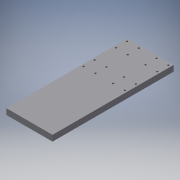
# Autodesk Inventor part: BLOCO_SUPORTE_EIXO_Z
Saved by Autodesk Inventor 2018 (Build 220112000, 112)
## iProperties
Created: 2018-10-10
Part Number: BLOCO_SUPORTE_EIXO_Z
Material: Genérico
Document SubType Name: Modeling
Designer: Georgines
Density: 1 g/cm^3
Appearance: Padrão
Author: Georgines
Autodesk Inventor part; units mm, degrees
ref_plane "YZ Plane" through (0, 0, 0) normal (1, 0, 0) x (0, 1, 0)
ref_plane "XZ Plane" through (0, 0, 0) normal (0, 1, 0) x (-1, 0, 0)
ref_plane "XY Plane" through (0, 0, 0) normal (0, 0, 1) x (1, 0, 0)
sketch "Esboço1" plane through (0, 0, 0) normal (0, 0, 1) x (1, 0, 0)
  line L0 (-20, 180.23) -> (105, 180.23)
  line L1 (105, 180.23) -> (105, -148.24)
  line L2 (105, -148.24) -> (-20, -148.24)
  line L3 (-20, -148.24) -> (-20, 180.23)
  dimension "d0" = 125
  dimension "d1" = 328.47
  constraints: 8 end point, 2 parallel, 1 horizontal, 1 perpendicular
  measures "d0" distance of L1.end L2.end
  measures "d1" distance of L0.end L1.end
extrude "Extrusão1" add sketch "Esboço1" along normal blind 15.88
sketch "Esboço3" plane through (0, 0, 0) normal (0, 0, -1) x (-1, 0, 0)
  circle A0 centre (-18.5, 54.73) radius 2.9 construction
  circle A1 centre (13.5, 54.73) radius 2.9 construction
  circle A2 centre (-66.5, 54.73) radius 2.9 construction
  circle A3 centre (-98.5, 54.73) radius 2.9 construction
  circle A4 centre (-98.5, 84.73) radius 2.9 construction
  circle A5 centre (-66.5, 84.73) radius 2.9 construction
  circle A6 centre (-18.5, 84.73) radius 2.9 construction
  circle A7 centre (13.5, 84.73) radius 2.9 construction
  circle A8 centre (-18.5, 172.73) radius 2.9 construction
  circle A9 centre (13.5, 172.73) radius 2.9 construction
  circle A10 centre (13.5, 142.73) radius 2.9 construction
  circle A11 centre (-18.5, 142.73) radius 2.9 construction
  circle A12 centre (-66.5, 172.73) radius 2.9 construction
  circle A13 centre (-98.5, 172.73) radius 2.9 construction
  circle A14 centre (-98.5, 142.73) radius 2.9 construction
  circle A15 centre (-66.5, 142.73) radius 2.9 construction
  point P0 (0, 0)
  constraints: 16 centre point
hole "Furo1" at (66.5, 142.73, 0) at (-13.5, 142.73, 0) at (18.5, 142.73, 0) at (-13.5, 172.73, 0) at (18.5, 172.73, 0) at (98.5, 142.73, 0) at (66.5, 172.73, 0) at (98.5, 172.73, 0) at (18.5, 84.73, 0) at (98.5, 84.73, 0) at (98.5, 54.73, 0) at (66.5, 54.73, 0) at (-13.5, 84.73, 0) at (18.5, 54.73, 0) at (-13.5, 54.73, 0) at (66.5, 84.73, 0) direction (0, 0, 1) diameter 5 end through all counterbore diameter 8 counterbore depth 6
